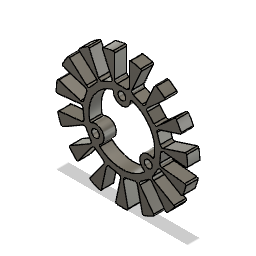
20221231_taiya_cover-5mm v1 (Autodesk Fusion 360 design; units mm, degrees)
Autodesk Fusion 360 part; units mm, degrees
sketch "スケッチ1" plane through (0, 0, 0) normal (0, 0, 1) x (1, 0, 0)
  arc A0 (16.0776, -5.8183) -> (14.7116, -6.1844) centre (15.5776, -6.6844) ccw
  arc A1 (12.8462, -23.7482) -> (13.0128, -23.0145) centre (12.6083, -23.3084) ccw
  arc A2 (15.537, -3.644) -> (16.427, -4.7431) centre (16.5315, -3.7486) ccw
  arc A3 (26.2441, -6.344) -> (25.8104, -5.7293) centre (25.7581, -6.2266) ccw
  line L0 (15.9551, 0.3341) -> (15.537, -3.644)
  line L1 (0.5653, -17.0887) -> (2.527, -26.3176)
  arc A4 (21.3948, -16.47) -> (21.2486, -15.732) centre (20.9986, -16.165) ccw
  arc A5 (12.4759, -3.1636) -> (13.2006, -2.8274) centre (12.7117, -2.7227) ccw
  arc A6 (18.6162, -19.556) -> (21.3948, -16.47) centre (0, 0) ccw
  line L2 (26.4375, 0.2378) -> (17.0542, 1.2241)
  arc A7 (26.4375, 0.2378) -> (26.9896, 0.749) centre (26.4898, 0.7351) ccw
  line L3 (14.7116, -6.1844) -> (12.7116, -9.6485)
  line L4 (16.427, -4.7431) -> (25.8104, -5.7293)
  arc A8 (2.0763, -26.92) -> (2.527, -26.3176) centre (2.0379, -26.4215) ccw
  arc A9 (24.2486, -10.5358) -> (24.9609, -10.2935) centre (24.4986, -10.1028) ccw
  arc A10 (12.7116, -9.6485) -> (13.0776, -11.0145) centre (13.5776, -10.1485) ccw
  arc A11 (24.9609, -10.2935) -> (26.2441, -6.344) centre (0, 0) ccw
  arc A12 (17.0542, 1.2241) -> (15.9551, 0.3341) centre (16.9497, 0.2295) ccw
  arc A13 (17.8669, -19.4878) -> (18.6162, -19.556) centre (18.2714, -19.1939) ccw
  line L5 (-12.7116, -9.6485) -> (-14.7116, -6.1844)
  arc A14 (-25.8104, -5.7293) -> (-26.2441, -6.344) centre (-25.7581, -6.2266) ccw
  line L6 (-6.4342, -15.8412) -> (-8.3958, -25.0701)
  arc A15 (-13.2006, -2.8274) -> (-12.4759, -3.1636) centre (-12.7117, -2.7227) ccw
  arc A16 (-7.467, -15.3814) -> (-7.6883, -13.9846) centre (-8.276, -14.7936) ccw
  arc A17 (-16.427, -4.7431) -> (-15.537, -3.644) centre (-16.5315, -3.7486) ccw
  line L7 (-7.6883, -13.9846) -> (-10.9243, -11.6334)
  line L8 (-16.0776, -5.8183) -> (-24.2486, -10.5358)
  arc A18 (-21.3948, -16.47) -> (-18.6162, -19.556) centre (0, 0) ccw
  arc A19 (-5.2481, -15.071) -> (-6.4342, -15.8412) centre (-5.456, -16.0492) ccw
  line L9 (-2.527, -26.3176) -> (-0.5653, -17.0887)
  line L10 (-25.8104, -5.7293) -> (-16.427, -4.7431)
  arc A20 (-18.6162, -19.556) -> (-17.8669, -19.4878) centre (-18.2714, -19.1939) ccw
  arc A21 (-8.9777, -9.2226) -> (-9.0489, -10.0183) centre (-8.7138, -9.6473) ccw
  line L11 (-12.3211, -11.8547) -> (-17.8669, -19.4878)
  arc A22 (-14.7116, -6.1844) -> (-16.0776, -5.8183) centre (-15.5776, -6.6844) ccw
  arc A23 (-12.8462, -23.7482) -> (-9.0525, -25.4372) centre (0, 0) ccw
  arc A24 (-13.0776, -11.0145) -> (-12.7116, -9.6485) centre (-13.5776, -10.1485) ccw
  arc A25 (-7.6279, 25.9001) -> (-7.9435, 25.2171) centre (-7.4867, 25.4205) ccw
  arc A26 (-3.566, 26.7635) -> (-7.6279, 25.9001) centre (0, 0) ccw
  arc A27 (-14.5166, 9.0339) -> (-13.1043, 9.1079) centre (-13.8475, 9.7771) ccw
  arc A28 (-3, 26.2679) -> (-3.566, 26.7635) centre (-3.5, 26.2679) ccw
  line L12 (-8.2669, 13.6505) -> (-4.6127, 15.2775)
  arc A29 (-14.1434, 22.9992) -> (-17.503, 20.5583) centre (0, 0) ccw
  arc A30 (-14.4399, 6.7947) -> (-15.0819, 8.0548) centre (-15.3909, 7.1037) ccw
  line L13 (-15.6759, 2.9905) -> (-14.4399, 6.7947)
  arc A31 (-4.6127, 15.2775) -> (-4.1059, 16.5978) centre (-5.0194, 16.191) ccw
  line L14 (-17.0542, 1.2241) -> (-26.4375, 0.2378)
  line L15 (-21.5282, 15.3472) -> (-14.5166, 9.0339)
  arc A32 (-16.936, 2.3485) -> (-15.6759, 2.9905) centre (-16.627, 3.2995) ccw
  arc A33 (-13.4247, 22.7767) -> (-14.1434, 22.9992) centre (-13.8815, 22.5733) ccw
  line L16 (-10.5018, 13.4928) -> (-17.5134, 19.8061)
  line L17 (-21.2486, -15.732) -> (-13.0776, -11.0145)
  line L18 (-13.0128, -23.0145) -> (-7.467, -15.3814)
  arc A34 (-26.2441, -6.344) -> (-24.9609, -10.2935) centre (0, 0) ccw
  arc A35 (-24.9609, -10.2935) -> (-24.2486, -10.5358) centre (-24.4986, -10.1028) ccw
  arc A36 (-0.5653, -17.0887) -> (-1.3355, -15.9027) centre (-1.5434, -16.8808) ccw
  line L19 (-1.3355, -15.9027) -> (-5.2481, -15.071)
  arc A37 (-10.9243, -11.6334) -> (-12.3211, -11.8547) centre (-11.5121, -12.4425) ccw
  arc A38 (-21.5282, 15.3472) -> (-22.2753, 15.2582) centre (-21.8628, 14.9756) ccw
  arc A39 (-22.2753, 15.2582) -> (-24.3516, 11.6619) centre (0, 0) ccw
  arc A40 (-24.3516, 11.6619) -> (-24.0552, 10.9704) centre (-23.9007, 11.4459) ccw
  arc A41 (-26.9896, 0.749) -> (-26.4375, 0.2378) centre (-26.4898, 0.7351) ccw
  arc A42 (-3.4982, 12.3863) -> (-4.1517, 12.8458) centre (-3.9979, 12.37) ccw
  arc A43 (-17.503, 20.5583) -> (-17.5134, 19.8061) centre (-17.1789, 20.1776) ccw
  arc A44 (8.2669, 13.6505) -> (9.5872, 14.1573) centre (8.6736, 14.5641) ccw
  arc A45 (-2.0763, -26.92) -> (2.0763, -26.92) centre (0, 0) ccw
  circle A46 centre (0, 12.5) radius 1.6
  arc A47 (24.0552, 10.9704) -> (24.3516, 11.6619) centre (23.9007, 11.4459) ccw
  line L20 (16.936, 2.3485) -> (25.9093, 5.264)
  arc A48 (22.2753, 15.2582) -> (21.5282, 15.3472) centre (21.8628, 14.9756) ccw
  arc A49 (3.566, 26.7635) -> (3, 26.2679) centre (3.5, 26.2679) ccw
  arc A50 (17.5134, 19.8061) -> (17.503, 20.5583) centre (17.1789, 20.1776) ccw
  arc A51 (10.5018, 13.4928) -> (10.4278, 12.0805) centre (11.171, 12.7496) ccw
  arc A52 (15.6759, 2.9905) -> (16.936, 2.3485) centre (16.627, 3.2995) ccw
  arc A53 (13.1043, 9.1079) -> (14.5166, 9.0339) centre (13.8475, 9.7771) ccw
  arc A54 (2, 15.8328) -> (3, 16.8328) centre (2, 16.8328) ccw
  arc A55 (26.5555, 4.8789) -> (25.9093, 5.264) centre (26.0638, 4.7885) ccw
  arc A56 (7.6279, 25.9001) -> (3.566, 26.7635) centre (0, 0) ccw
  line L21 (-15.537, -3.644) -> (-15.9551, 0.3341)
  arc A57 (-4.1517, 12.8458) -> (-13.2006, -2.8274) centre (0, 0) ccw
  arc A58 (-15.9551, 0.3341) -> (-17.0542, 1.2241) centre (-16.9497, 0.2295) ccw
  arc A59 (-25.9093, 5.264) -> (-26.5555, 4.8789) centre (-26.0638, 4.7885) ccw
  line L22 (-13.4247, 22.7767) -> (-9.5872, 14.1573)
  line L23 (-4.1059, 16.5978) -> (-7.9435, 25.2171)
  arc A60 (-26.5555, 4.8789) -> (-26.9896, 0.749) centre (0, 0) ccw
  line L24 (-25.9093, 5.264) -> (-16.936, 2.3485)
  arc A61 (-3, 16.8328) -> (-2, 15.8328) centre (-2, 16.8328) ccw
  line L25 (-15.0819, 8.0548) -> (-24.0552, 10.9704)
  line L26 (-3, 26.2679) -> (-3, 16.8328)
  arc A62 (-10.4278, 12.0805) -> (-10.5018, 13.4928) centre (-11.171, 12.7496) ccw
  arc A63 (-9.5872, 14.1573) -> (-8.2669, 13.6505) centre (-8.6736, 14.5641) ccw
  line L27 (-13.1043, 9.1079) -> (-10.4278, 12.0805)
  arc A64 (-21.2486, -15.732) -> (-21.3948, -16.47) centre (-20.9986, -16.165) ccw
  arc A65 (-13.0128, -23.0145) -> (-12.8462, -23.7482) centre (-12.6083, -23.3084) ccw
  circle A66 centre (-10.8253, -6.25) radius 1.6
  arc A67 (-9.0525, -25.4372) -> (-8.3958, -25.0701) centre (-8.8849, -24.9661) ccw
  arc A68 (-2.527, -26.3176) -> (-2.0763, -26.92) centre (-2.0379, -26.4215) ccw
  line L28 (3, 16.8328) -> (3, 26.2679)
  arc A69 (6.4342, -15.8412) -> (5.2481, -15.071) centre (5.456, -16.0492) ccw
  line L29 (5.2481, -15.071) -> (1.3355, -15.9027)
  arc A70 (8.3958, -25.0701) -> (9.0525, -25.4372) centre (8.8849, -24.9661) ccw
  arc A71 (17.503, 20.5583) -> (14.1434, 22.9992) centre (0, 0) ccw
  arc A72 (9.0525, -25.4372) -> (12.8462, -23.7482) centre (0, 0) ccw
  arc A73 (14.1434, 22.9992) -> (13.4247, 22.7767) centre (13.8815, 22.5733) ccw
  line L30 (8.3958, -25.0701) -> (6.4342, -15.8412)
  line L31 (14.4399, 6.7947) -> (15.6759, 2.9905)
  line L32 (24.0552, 10.9704) -> (15.0819, 8.0548)
  arc A74 (4.1517, 12.8458) -> (3.4982, 12.3863) centre (3.9979, 12.37) ccw
  arc A75 (9.0489, -10.0183) -> (8.9777, -9.2226) centre (8.7138, -9.6473) ccw
  line L33 (24.2486, -10.5358) -> (16.0776, -5.8183)
  arc A76 (26.9896, 0.749) -> (26.5555, 4.8789) centre (0, 0) ccw
  arc A77 (13.2006, -2.8274) -> (4.1517, 12.8458) centre (0, 0) ccw
  line L34 (17.5134, 19.8061) -> (10.5018, 13.4928)
  line L35 (7.467, -15.3814) -> (13.0128, -23.0145)
  arc A78 (1.3355, -15.9027) -> (0.5653, -17.0887) centre (1.5434, -16.8808) ccw
  arc A79 (15.0819, 8.0548) -> (14.4399, 6.7947) centre (15.3909, 7.1037) ccw
  arc A80 (-9.0489, -10.0183) -> (9.0489, -10.0183) centre (0, 0) ccw
  arc A81 (12.3211, -11.8547) -> (10.9243, -11.6334) centre (11.5121, -12.4425) ccw
  circle A82 centre (10.8253, -6.25) radius 1.6
  line L36 (-2, 15.8328) -> (2, 15.8328)
  arc A83 (4.1059, 16.5978) -> (4.6127, 15.2775) centre (5.0194, 16.191) ccw
  line L37 (7.9435, 25.2171) -> (4.1059, 16.5978)
  line L38 (9.5872, 14.1573) -> (13.4247, 22.7767)
  arc A84 (24.3516, 11.6619) -> (22.2753, 15.2582) centre (0, 0) ccw
  line L39 (4.6127, 15.2775) -> (8.2669, 13.6505)
  line L40 (17.8669, -19.4878) -> (12.3211, -11.8547)
  line L41 (14.5166, 9.0339) -> (21.5282, 15.3472)
  arc A85 (7.9435, 25.2171) -> (7.6279, 25.9001) centre (7.4867, 25.4205) ccw
  line L42 (10.4278, 12.0805) -> (13.1043, 9.1079)
  arc A86 (7.6883, -13.9846) -> (7.467, -15.3814) centre (8.276, -14.7936) ccw
  line L43 (10.9243, -11.6334) -> (7.6883, -13.9846)
  line L44 (13.0776, -11.0145) -> (21.2486, -15.732)
  arc A87 (-3.4982, 12.3863) -> (3.4982, 12.3863) centre (0, 12.5) ccw
  arc A88 (-8.9777, -9.2226) -> (-12.4759, -3.1636) centre (-10.8253, -6.25) ccw
  arc A89 (12.4759, -3.1636) -> (8.9777, -9.2226) centre (10.8253, -6.25) ccw
  point P0 (3, 15.8328)
  point P1 (3, 26.8328)
  dimension "d4" = 360
  dimension "d5" = 54
  dimension "d7" = 6
  dimension "d8" = 11
  dimension "d9" = 1
  dimension "d10" = 1
  dimension "d41" = 0.5
  dimension "d42" = 0.5
  dimension "d43" = 0.5
  dimension "d44" = 0.5
  dimension "d45" = 0.5
  dimension "d46" = 0.5
  dimension "d47" = 0.5
  dimension "d48" = 0.5
  dimension "d49" = 0.5
  dimension "d50" = 0.5
  dimension "d51" = 0.5
  dimension "d52" = 0.5
  dimension "d53" = 0.5
  dimension "d54" = 0.5
  dimension "d55" = 0.5
  dimension "d56" = 0.5
  dimension "d59" = 0.5
  dimension "d60" = 0.5
  dimension "d61" = 0.5
  dimension "d62" = 0.5
  dimension "d63" = 0.5
  dimension "d64" = 0.5
  dimension "d65" = 0.5
  dimension "d66" = 0.5
  dimension "d67" = 0.5
  dimension "d68" = 0.5
  dimension "d69" = 0.5
  dimension "d70" = 0.5
  dimension "d71" = 3.2
  dimension "d75" = 0.5
  dimension "d76" = 0.5
  dimension "d82" = 7
  dimension "d84" = 360
  constraint coincident A6.centre A11.centre
  constraint vertical L26
  constraint perpendicular L26 L36
  constraint perpendicular L28 L36
  constraint tangent A61 L26
  constraint tangent A61 L36
  constraint coincident P0 L36
  constraint coincident P0 L28
  constraint tangent A54 L36
  constraint tangent A54 L28
  constraint concentric A26 A56
  constraint concentric A26 A71
  constraint concentric A26 A84
  constraint concentric A26 A76
  constraint concentric A11 A26
  constraint concentric A6 A26
  constraint concentric A26 A72
  constraint concentric A23 A26
  constraint concentric A18 A26
  constraint concentric A26 A34
  constraint concentric A26 A60
  constraint concentric A26 A39
  constraint concentric A26 A29
  constraint tangent A28 L26
  constraint tangent A26 A28
  constraint coincident P1 L28
  constraint coincident P1 A56
  constraint tangent A49 L28
  constraint tangent A49 A56
  constraint tangent L37 A85
  constraint tangent A56 A85
  constraint tangent A25 L23
  constraint tangent A25 A26
  constraint tangent A33 L22
  constraint tangent A29 A33
  constraint tangent L16 A43
  constraint tangent A29 A43
  constraint tangent A73 L38
  constraint tangent A71 A73
  constraint tangent A50 L34
  constraint tangent A50 A71
  constraint tangent A48 L41
  constraint tangent A48 A84
  constraint tangent A47 L32
  constraint tangent A47 A84
  constraint tangent L20 A55
  constraint tangent A55 A76
  constraint tangent L2 A7
  constraint tangent A7 A76
  constraint tangent L15 A38
  constraint tangent A38 A39
  constraint tangent A40 L25
  constraint tangent A39 A40
  constraint tangent A59 L24
  constraint tangent A59 A60
  constraint tangent L14 A41
  constraint tangent A41 A60
  constraint tangent A14 L10
  constraint tangent A14 A34
  constraint tangent L8 A35
  constraint tangent A34 A35
  constraint tangent A3 L4
  constraint tangent A3 A11
  constraint tangent A9 L33
  constraint tangent A9 A11
  constraint tangent A4 L44
  constraint tangent A4 A6
  constraint tangent A13 L40
  constraint tangent A6 A13
  constraint tangent A1 L35
  constraint tangent A1 A72
  constraint tangent A70 L30
  constraint tangent A70 A72
  constraint tangent L18 A65
  constraint tangent A23 A65
  constraint tangent L6 A67
  constraint tangent A23 A67
  constraint tangent L17 A64
  constraint tangent A18 A64
  constraint tangent A20 L11
  constraint tangent A18 A20
  constraint concentric A29 A57
  constraint tangent A42 A57
  constraint tangent A57 A74
  constraint concentric A57 A77
  constraint concentric A57 A80
  constraint concentric A46 A87
  measures "d5" diameter of A26
  measures "d7" distance of L26 L28
  measures "d8" distance of P0 P1
  measures "d9" radius of A61
  measures "d10" radius of A54
  measures "d41" radius of A28
  measures "d42" radius of A49
  measures "d43" radius of A85
  measures "d44" radius of A25
  measures "d45" radius of A33
  measures "d46" radius of A43
  measures "d47" radius of A73
  measures "d48" radius of A50
  measures "d49" radius of A48
  measures "d50" radius of A47
  measures "d51" radius of A55
  measures "d52" radius of A7
  measures "d53" radius of A38
  measures "d54" radius of A40
  measures "d55" radius of A59
  measures "d56" radius of A41
  measures "d59" radius of A14
  measures "d60" radius of A35
  measures "d61" radius of A3
  measures "d62" radius of A9
  measures "d63" radius of A4
  measures "d64" radius of A13
  measures "d65" radius of A1
  measures "d66" radius of A70
  measures "d67" radius of A65
  measures "d68" radius of A67
  measures "d69" radius of A64
  measures "d70" radius of A20
  measures "d71" diameter of A46
  measures "d75" radius of A42
  measures "d76" radius of A74
  measures "d82" diameter of A87
extrude "押し出し1" add sketch "スケッチ1" along normal blind 5
